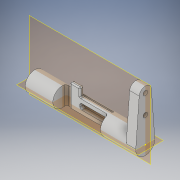
# Autodesk Inventor part: SR-T-07
Saved by Autodesk Inventor 2019.4 (Build 234330000, 330)
## iProperties
Created: 2019-06-15
Part Number: SR-T-07
Material: 一般
Document SubType Name: Modeling
Designer: Koki Shinjo
Mass: 0.515991 g
Surface Area: 7.04675 cm^2
Volume: 0.515991 cm^3
Density: 1 g/cm^3
Appearance: 既定
Author: Koki Shinjo
Autodesk Inventor part; units mm, degrees
ref_plane "YZ Plane" through (0, 0, 0) normal (1, 0, 0) x (0, 1, 0)
ref_plane "XY Plane" through (0, 0, 0) normal (0, 0, 1) x (1, 0, 0)
sketch "スケッチ1" plane through (0, 0, 0) normal (0, 0, 1) x (1, 0, 0)
  line L0 (0, 0) -> (0, 2.5)
  line L1 (0, 2.5) -> (-29, 2.5)
  line L2 (-29, 2.5) -> (-29, 0)
  line L3 (-29, 0) -> (0, 0)
  dimension "d0" = 29
  dimension "d1" = 2.5
  constraints: 8 end point, 3 perpendicular, 1 vertical
  measures "d0" distance of L0.end L1.end
  measures "d1" distance of L0.start L0.end
revolve "回転1" add sketch "スケッチ1" angle 360 about axis through (-29, 0, 0) along (1, 0, 0)
sketch "スケッチ2" plane through (0, 0, 0) normal (1, 0, 0) x (0, 0, -1)
  circle A0 centre (0, 6.7) radius 0.6
  circle A1 centre (0, 11.7) radius 0.6
  circle A2 centre (0, 11.7) radius 1.6
  line L0 (-1.5953, 11.8231) -> (-2.4926, 0.1923)
  circle A3 centre (0, 0) radius 2.5 projected
  line L1 (2.4926, 0.1923) -> (1.5953, 11.8231)
  dimension "d3" = 1.2
  dimension "d4" = 5
  dimension "d5" = 6.7
  dimension "d6" = 3.2
  constraints: 4 end point, 4 point on circle, 4 tangent, 3 centre point, 2 vertical alignment, 1 coincident, 1 equal radius
  measures "d3" diameter of A1
  measures "d4" distance of A1.centre A0.centre
  measures "d5" distance of point (0, 0) A0.centre
  measures "d6" diameter of A2
extrude "押し出し1" add sketch "スケッチ2" against normal blind 2.5 contours A2 | A2 L1 A3 L0
ref_plane "作業平面1" through (0, 0, 0) normal (0, 1, 0) x (-1, 0, 0)
sketch "スケッチ3" plane through (0, 0, 0) normal (0, 1, 0) x (-1, 0, 0)
  line L0 (0, 1.5953) -> (0, 2.4926) construction
  line L1 (0, 1.5953) -> (2.5, 1.5953) construction
  line L2 (2.5, 2.4926) -> (2.5, 1.5953) construction
  line L3 (2.5, 2.4926) -> (0, 2.4926) construction
  line L4 (0, 0.6) -> (2.5, 0.6) construction
  line L5 (0, 1.5953) -> (0, -1.5953) construction
  line L6 (0, -2.4926) -> (0, -1.5953) construction
  point P0 (0, 0)
sketch "スケッチ4" plane through (0, 0, 0) normal (0, 0, 1) x (1, 0, 0)
  line L0 (-29, 2.5) -> (-2.5, 2.5) projected
  line L1 (-19.2495, 2.5) -> (-16.6495, 2.5)
  line L2 (-16.6495, 2.5) -> (-16.6495, 4.8)
  line L3 (-16.6495, 4.8) -> (-19.2495, 4.8)
  line L4 (-19.2495, 4.8) -> (-19.2495, 2.5)
  line L5 (-19.4495, 3.871) -> (-14.8405, 3.871) construction
  line L6 (-19.4495, 4.8) -> (-19.4495, 3.871) construction
  line L7 (-19.4495, 4.8) -> (-16.4495, 4.8) construction
  line L8 (-16.4495, 4.8) -> (-14.8405, 3.871) construction
  line L9 (-16.6495, 2.5) -> (-19.2495, 2.5)
  line L10 (-19.2495, 2.5) -> (-19.2495, 1.5)
  line L11 (-19.2495, 1.5) -> (-16.6495, 1.5)
  line L12 (-16.6495, 1.5) -> (-16.6495, 2.5)
  point P0 (0, 0)
  dimension "d10" = 0.2
  dimension "d11" = 0
  dimension "d12" = 0.2
  dimension "d13" = 1
  constraints: 16 end point, 4 parallel, 2 horizontal, 2 perpendicular, 1 point on line
  measures "d10" distance between parallel lines of L6 L4
  measures "d11" distance between parallel lines of L7 L3
  measures "d12" distance from line of L7.end L2
  measures "d13" distance of L1.start L10.end
extrude "押し出し2" add sketch "スケッチ4" along normal mid plane 1
fillet "フィレット1" radius 0.5 2 edges at (-19.2495, 4.8, 0) (-16.6495, 4.8, 0)
fillet "フィレット2" radius 0.5 2 edges at (-16.6495, 2.4873, -0.2513) (-16.6495, 2.4873, 0.2513)
sketch "スケッチ5" plane through (-18.7495, 4.8, -0.5) normal (0, 1, 0) x (1, 0, 0)
  line L0 (0, -1) -> (-0.5, -1) projected
  line L1 (-0.5, -1) -> (9.5, -1)
  line L2 (9.5, -1) -> (9.5, 0) construction
  line L3 (9.5, 0) -> (-0.5, 0)
  line L4 (-0.5, 0) -> (-0.5, -1)
  line L5 (-0.5, 0) -> (0, 0) projected
  line L6 (10, -1.5) -> (-1, -1.5)
  line L7 (-1, -1.5) -> (-1, 0.5)
  line L8 (-1, 0.5) -> (10, 0.5)
  line L9 (10, 0.5) -> (10, -1.5) construction
  line L10 (9.5, -1) -> (9.5, -1.5)
  line L11 (9.5, 0) -> (9.5, 0.5)
  point P0 (18.7495, -0.5)
  dimension "d18" = 10
  dimension "d19" = 0.5
  constraints: 20 end point, 4 parallel, 4 point on line, 3 perpendicular, 1 horizontal, 3 other
  measures "d18" distance of L2.end L3.end
  measures "d19" distance between parallel lines of L1 L6
extrude "押し出し3" cut sketch "スケッチ5" against normal up to next
ref_plane "作業平面2" through (0, 0, 0) normal (0, 0, 1) x (1, 0, 0)
sketch "スケッチ6" plane through (0, 0, 0) normal (0, 0, 1) x (1, 0, 0)
  line L0 (-9.2495, 2.4495) -> (-16.1495, 2.4495) construction
  line L1 (-16.1495, 2.4495) -> (-16.1495, 2.4495) construction
  line L2 (-16.1495, 2.4495) -> (-9.2495, 2.4495) construction
  line L3 (-9.2495, 2.4495) -> (-9.2495, 2.2913) construction
  line L4 (-9.2495, 2.2913) -> (-19.7495, 2.2913) construction
  line L5 (-19.7495, 2.2913) -> (-19.7495, 2.2913) construction
  line L6 (-19.7495, 2.2913) -> (-9.2495, 2.2913) construction
  line L7 (-9.2495, 2.2913) -> (-9.2495, 2.4495) construction
  line L8 (-19.2495, -2.4495) -> (-19.2495, -2.4495) construction
  line L9 (-19.2495, -2.4495) -> (-9.2495, -2.4495) construction
  line L10 (-9.2495, -2.4495) -> (-9.2495, -2.2913) construction
  line L11 (-9.2495, -2.2913) -> (-19.7495, -2.2913) construction
  line L12 (-19.7495, -2.2913) -> (-19.7495, -2.2913) construction
  line L13 (-19.7495, -2.2913) -> (-9.2495, -2.2913) construction
  line L14 (-9.2495, -2.2913) -> (-9.2495, -2.4495) construction
  line L15 (-9.2495, -2.4495) -> (-19.2495, -2.4495) construction
  line L16 (-2.5, 0.1923) -> (0, 0.1923) construction
  line L17 (-2.5, 0.1923) -> (-2.5, 0.1923) construction
  line L18 (-2.5, 0.1923) -> (0, 0.1923) construction
  line L19 (0, 0.1923) -> (0, 0.1923) construction
  line L20 (-29, -2.5) -> (-29, 2.5) construction
  line L21 (-9.2495, -2.4495) -> (-19.2495, -2.4495) construction
  line L22 (-9.2495, 2.4495) -> (-9.2495, -2.4495) construction
  line L23 (-16.1495, 2.4495) -> (-9.2495, 2.4495) construction
  line L24 (-16.6495, 2.958) -> (-16.6495, 4.3) construction
  arc A0 (-16.6495, 4.3) -> (-17.1495, 4.8) centre (-17.1495, 4.3) ccw construction
  line L25 (-17.1495, 4.8) -> (-18.7495, 4.8) construction
  arc A1 (-18.7495, 4.8) -> (-19.2495, 4.3) centre (-18.7495, 4.3) ccw construction
  line L26 (-19.2495, 4.3) -> (-19.2495, -2.4495) construction
  line L27 (-19.2495, -2.5) -> (-19.2495, -2.4495) projected
  line L28 (-19.2495, -2.5) -> (-9.2495, -2.5)
  line L29 (-9.2495, -2.5) -> (-9.2495, -1)
  line L30 (-9.2495, -1) -> (-19.2495, -1)
  line L31 (-19.2495, -1) -> (-19.2495, -2.5)
  line L32 (-9.2495, 1.5) -> (-16.6495, 1.5)
  line L33 (-16.6495, 1.5) -> (-16.6495, 0)
  line L34 (-16.6495, 0) -> (-9.2495, 0)
  line L35 (-9.2495, 0) -> (-9.2495, 1.5)
  line L36 (-29, 2.5) -> (-2.5, 2.5) construction
  point P0 (0, 0)
  dimension "d22" = 1.5
  dimension "d23" = 1
  dimension "d24" = 1
  constraints: 16 end point, 4 parallel, 3 point on line, 2 horizontal, 2 perpendicular, 1 other
  measures "d22" distance between parallel lines of L28 L30
  measures "d23" distance between parallel lines of L32 L36
  measures "d24" distance between parallel lines of L30 L34
extrude "押し出し4" cut sketch "スケッチ6" along normal mid plane 1
fillet "フィレット3" radius 0.5 6 edges at (-9.2495, 0, 0) (-9.2495, 1.5, 0) (-9.2495, -1, 0) (-16.6495, 0, 0) (-16.6495, 1.5, 0) (-19.2495, -1, 0)
move faces "移動1" translate (-2, 0, 0) faces at (-19.7495, 0.8255, 0.114)
delete faces "削除1" heal yes whole lump no faces at (-17.1121, 4.7986, 0.1667) (-18.7869, 4.7986, 0.1667)
fillet "フィレット4" radius 0.3 2 edges at (-17.9495, 4.8, 0.5) (-17.9495, 4.8, -0.5)
delete faces "削除2" heal yes whole lump no faces at (-16.648, 2.9398, 0.352)
delete faces "削除3" heal yes whole lump no faces at (-19.1825, -0.75, 0.1667)
delete faces "削除4" heal yes whole lump no faces at (-9.4995, -1.067, 0.1667)
fillet "フィレット5" radius 0.3 10 edges at (-16.6495, 4.7121, -0.4121) (-16.6495, 3.4747, -0.5) (-16.6495, 4.7121, 0.4121) (-16.6495, 3.4747, 0.5) (-16.6495, 4.8, 0) (-19.2495, 1.75, 0.5) (-19.2495, 4.8, 0) (-19.2495, 4.7121, -0.4121) (-19.2495, 1.75, -0.5) (-19.2495, 4.7121, 0.4121)
fillet "フィレット6" radius 0.3 4 edges at (-16.7391, 2.4655, 0.4138) (-16.7391, 2.4655, -0.4138) (-16.6495, 2.498, -0.1001) (-16.6495, 2.498, 0.1001)
fillet "フィレット7" radius 0.3 1 edges at (-9.2495, -1, 0)
delete faces "削除5" heal yes whole lump no faces at (-17.5828, -0.7638, 1)
fillet "フィレット8" radius 0.5 1 edges at (-21.7495, 0, -1)
fillet "フィレット9" radius 0.5 2 edges at (-9.2495, 1.7247, 0.5) (-9.2495, -0.4, 0.5)
